Autodesk Fusion 360 part; units mm, degrees
(part 7 of 14)
  arc A1856 (48.735, 36.8717) -> (48.735, 37.1384) centre (48.735, 37.005) ccw
  line L3081 (47.395, 52.0775) -> (47.395, 54.3505)
  line L3082 (46.395, 46.3495) -> (46.395, 48.6225)
  line L3083 (46.895, 52.0775) -> (46.895, 54.3505)
  line L3084 (17.461, 23.167) -> (27.461, 23.167)
  line L3085 (27.461, 13.167) -> (17.461, 13.167)
  arc A1857 (52.735, 36.8717) -> (52.735, 37.1384) centre (52.735, 37.005) ccw
  line L3086 (17.461, 13.167) -> (17.461, 23.167)
  line L3087 (61.3283, 55.098) -> (60.4393, 55.098)
  arc A1858 (16.7662, 22.5764) -> (17.1475, 22.5764) centre (16.9568, 22.5764) ccw
  arc A1859 (17.1475, 22.5764) -> (16.7662, 22.5764) centre (16.9568, 22.5764) ccw
  line L3088 (27.461, 23.167) -> (27.461, 13.167)
  arc A1860 (50.735, 37.1384) -> (50.735, 36.8717) centre (50.735, 37.005) ccw
  line L3089 (46.395, 46.3495) -> (46.395, 48.6225)
  line L3090 (46.895, 46.3495) -> (46.895, 48.6225)
  line L3091 (47.395, 46.3495) -> (47.395, 48.6225)
  line L3092 (47.895, 46.3495) -> (47.895, 48.6225)
  arc A1861 (51.735, 36.8717) -> (51.735, 37.1384) centre (51.735, 37.005) ccw
  arc A1862 (49.735, 36.8717) -> (49.735, 37.1384) centre (49.735, 37.005) ccw
  arc A1863 (52.735, 36.8717) -> (52.735, 37.1384) centre (52.735, 37.005) ccw
  arc A1864 (50.735, 36.8717) -> (50.735, 37.1384) centre (50.735, 37.005) ccw
  arc A1865 (51.735, 37.1384) -> (51.735, 36.8717) centre (51.735, 37.005) ccw
  arc A1866 (48.735, 36.8717) -> (48.735, 37.1384) centre (48.735, 37.005) ccw
  arc A1867 (52.735, 36.8717) -> (52.735, 37.1384) centre (52.735, 37.005) ccw
  arc A1868 (50.735, 37.1384) -> (50.735, 36.8717) centre (50.735, 37.005) ccw
  arc A1869 (51.735, 36.8717) -> (51.735, 37.1384) centre (51.735, 37.005) ccw
  arc A1870 (51.735, 37.1384) -> (51.735, 36.8717) centre (51.735, 37.005) ccw
  arc A1871 (51.735, 37.1384) -> (51.735, 36.8717) centre (51.735, 37.005) ccw
  arc A1872 (50.735, 37.1384) -> (50.735, 36.8717) centre (50.735, 37.005) ccw
  arc A1873 (48.735, 37.1384) -> (48.735, 36.8717) centre (48.735, 37.005) ccw
  arc A1874 (52.735, 37.1384) -> (52.735, 36.8717) centre (52.735, 37.005) ccw
  line L3093 (47.395, 52.0775) -> (47.395, 54.3505)
  line L3094 (47.895, 52.0775) -> (47.895, 54.3505)
  line L3095 (46.895, 46.3495) -> (46.895, 48.6225)
  line L3096 (47.395, 46.3495) -> (47.395, 48.6225)
  arc A1875 (50.735, 36.8717) -> (50.735, 37.1384) centre (50.735, 37.005) ccw
  line L3097 (47.895, 46.3495) -> (47.895, 48.6225)
  arc A1876 (49.735, 37.1384) -> (49.735, 36.8717) centre (49.735, 37.005) ccw
  line L3098 (46.895, 52.0775) -> (46.895, 54.3505)
  line L3099 (46.895, 46.3495) -> (46.895, 48.6225)
  line L3100 (47.895, 52.0775) -> (47.895, 54.3505)
  arc A1877 (49.735, 36.8717) -> (49.735, 37.1384) centre (49.735, 37.005) ccw
  line L3101 (47.27, 11.525) -> (45.492, 11.525)
  line L3102 (9.7348, 30.754) -> (9.7348, 30.246)
  line L3103 (0.0248, 38.77) -> (0.0248, 25.27)
  line L3104 (9.4808, 30.5) -> (9.9888, 30.5)
  line L3105 (-5.0452, 28.845) -> (-3.9452, 27.745)
  line L3106 (51.715, 9.112) -> (51.715, 15.081)
  line L3107 (47.905, 15.081) -> (47.905, 9.112)
  line L3108 (47.27, 9.112) -> (47.27, 15.081)
  line L3109 (47.27, 14.065) -> (45.492, 14.065)
  line L3110 (9.4808, 30.5) -> (9.9888, 30.5)
  arc A1878 (9.7348, 30.7477) -> (9.7348, 30.2524) centre (9.7348, 30.5) ccw
  line L3111 (-5.2752, 25.77) -> (4.9948, 25.77)
  line L3112 (9.7348, 30.754) -> (9.7348, 30.246)
  arc A1879 (9.7348, 30.2524) -> (9.7348, 30.7477) centre (9.7348, 30.5) ccw
  line L3113 (50.445, 9.747) -> (50.445, 10.382)
  line L3114 (51.715, 15.081) -> (47.905, 15.081)
  line L3115 (54.128, 11.525) -> (52.35, 11.525)
  arc A1880 (9.7348, 30.2524) -> (9.7348, 30.7477) centre (9.7348, 30.5) ccw
  line L3116 (54.128, 11.525) -> (52.35, 11.525)
  line L3117 (54.128, 12.795) -> (52.35, 12.795)
  line L3118 (9.7348, 30.754) -> (9.7348, 30.246)
  line L3119 (52.35, 15.081) -> (52.35, 9.112)
  line L3120 (49.81, 9.112) -> (47.27, 9.112)
  line L3121 (47.27, 14.065) -> (45.492, 14.065)
  line L3122 (9.4808, 30.5) -> (9.9888, 30.5)
  line L3123 (47.27, 15.081) -> (52.35, 15.081)
  line L3124 (13.0848, 25.77) -> (13.0848, 37.77)
  line L3125 (9.7348, 30.754) -> (9.7348, 30.246)
  line L3126 (52.35, 9.112) -> (49.81, 9.112)
  line L3127 (47.905, 9.112) -> (51.715, 9.112)
  arc A1881 (9.7348, 30.7477) -> (9.7348, 30.2524) centre (9.7348, 30.5) ccw
  line L3128 (4.7648, 37.77) -> (-5.2752, 37.77)
  line L3129 (47.27, 11.525) -> (45.492, 11.525)
  arc A1882 (9.7348, 30.2524) -> (9.7348, 30.7477) centre (9.7348, 30.5) ccw
  arc A1883 (9.7348, 30.2524) -> (9.7348, 30.7477) centre (9.7348, 30.5) ccw
  line L3130 (54.128, 10.255) -> (52.35, 10.255)
  line L3131 (54.128, 11.525) -> (52.35, 11.525)
  line L3132 (54.128, 10.255) -> (52.35, 10.255)
  line L3133 (51.715, 9.747) -> (50.445, 9.747)
  line L3134 (54.128, 12.795) -> (52.35, 12.795)
  line L3135 (51.715, 9.112) -> (51.715, 15.081)
  line L3136 (50.445, 10.382) -> (51.715, 10.382)
  line L3137 (54.128, 14.065) -> (52.35, 14.065)
  line L3138 (54.128, 10.255) -> (52.35, 10.255)
  arc A1884 (9.7348, 30.7477) -> (9.7348, 30.2524) centre (9.7348, 30.5) ccw
  arc A1885 (53.747, 8.477) -> (52.985, 8.477) centre (53.366, 8.477) ccw
  line L3139 (54.128, 12.795) -> (52.35, 12.795)
  line L3140 (47.27, 11.525) -> (45.492, 11.525)
  arc A1886 (9.7348, 30.2524) -> (9.7348, 30.7477) centre (9.7348, 30.5) ccw
  arc A1887 (9.7348, 30.7477) -> (9.7348, 30.2524) centre (9.7348, 30.5) ccw
  line L3141 (-5.2752, 37.77) -> (-5.2752, 25.77)
  line L3142 (54.128, 14.065) -> (52.35, 14.065)
  line L3143 (-3.9452, 27.745) -> (-5.1452, 26.545)
  line L3144 (9.7348, 30.754) -> (9.7348, 30.246)
  arc A1888 (9.7348, 30.7477) -> (9.7348, 30.2524) centre (9.7348, 30.5) ccw
  line L3145 (47.27, 10.255) -> (45.492, 10.255)
  arc A1889 (9.7348, 30.2524) -> (9.7348, 30.7477) centre (9.7348, 30.5) ccw
  line L3146 (47.27, 14.065) -> (45.492, 14.065)
  line L3147 (9.4808, 30.5) -> (9.9888, 30.5)
  line L3148 (9.4808, 30.5) -> (9.9888, 30.5)
  arc A1890 (52.985, 8.477) -> (53.747, 8.477) centre (53.366, 8.477) ccw
  line L3149 (47.27, 12.795) -> (45.492, 12.795)
  line L3150 (54.128, 14.065) -> (52.35, 14.065)
  arc A1891 (9.7348, 30.7477) -> (9.7348, 30.2524) centre (9.7348, 30.5) ccw
  line L3151 (9.7348, 30.754) -> (9.7348, 30.246)
  arc A1892 (10.1158, 30.5) -> (9.3538, 30.5) centre (9.7348, 30.5) ccw
  arc A1893 (9.3538, 30.5) -> (10.1158, 30.5) centre (9.7348, 30.5) ccw
  arc A1894 (9.7348, 33.2476) -> (9.7348, 32.7523) centre (9.7348, 33) ccw
  line L3152 (9.4808, 33) -> (9.9888, 33)
  arc A1895 (9.7348, 33.2476) -> (9.7348, 32.7523) centre (9.7348, 33) ccw
  arc A1896 (9.7348, 30.7477) -> (9.7348, 30.2524) centre (9.7348, 30.5) ccw
  arc A1897 (9.7348, 30.7477) -> (9.7348, 30.2524) centre (9.7348, 30.5) ccw
  line L3153 (47.27, 12.795) -> (45.492, 12.795)
  arc A1898 (9.7348, 33.2476) -> (9.7348, 32.7523) centre (9.7348, 33) ccw
  line L3154 (47.27, 10.255) -> (45.492, 10.255)
  arc A1899 (9.7348, 32.7523) -> (9.7348, 33.2476) centre (9.7348, 33) ccw
  arc A1900 (9.7348, 30.2524) -> (9.7348, 30.7477) centre (9.7348, 30.5) ccw
  line L3155 (9.4808, 30.5) -> (9.9888, 30.5)
  arc A1901 (9.7348, 32.7523) -> (9.7348, 33.2476) centre (9.7348, 33) ccw
  line L3156 (9.4808, 33) -> (9.9888, 33)
  arc A1902 (9.7348, 32.7523) -> (9.7348, 33.2476) centre (9.7348, 33) ccw
  arc A1903 (9.7348, 32.7523) -> (9.7348, 33.2476) centre (9.7348, 33) ccw
  line L3157 (9.7348, 33.254) -> (9.7348, 32.746)
  line L3158 (9.7348, 30.754) -> (9.7348, 30.246)
  line L3159 (9.4808, 33) -> (9.9888, 33)
  line L3160 (47.27, 12.795) -> (45.492, 12.795)
  line L3161 (9.7348, 30.754) -> (9.7348, 30.246)
  line L3162 (4.7648, 25.77) -> (13.0848, 25.77)
  arc A1904 (9.7348, 33.2476) -> (9.7348, 32.7523) centre (9.7348, 33) ccw
  line L3163 (9.7348, 33.254) -> (9.7348, 32.746)
  arc A1905 (9.7348, 30.7477) -> (9.7348, 30.2524) centre (9.7348, 30.5) ccw
  line L3164 (9.7348, 33.254) -> (9.7348, 32.746)
  arc A1906 (9.7348, 30.2524) -> (9.7348, 30.7477) centre (9.7348, 30.5) ccw
  arc A1907 (9.7348, 30.2524) -> (9.7348, 30.7477) centre (9.7348, 30.5) ccw
  arc A1908 (10.1158, 30.5) -> (9.3538, 30.5) centre (9.7348, 30.5) ccw
  arc A1909 (9.7348, 33.2476) -> (9.7348, 32.7523) centre (9.7348, 33) ccw
  line L3165 (9.4808, 30.5) -> (9.9888, 30.5)
  line L3166 (9.4808, 33) -> (9.9888, 33)
  arc A1910 (9.7348, 33.2476) -> (9.7348, 32.7523) centre (9.7348, 33) ccw
  arc A1911 (9.7348, 33.2476) -> (9.7348, 32.7523) centre (9.7348, 33) ccw
  line L3167 (9.4808, 33) -> (9.9888, 33)
  arc A1912 (9.3538, 30.5) -> (10.1158, 30.5) centre (9.7348, 30.5) ccw
  line L3168 (9.4808, 30.5) -> (9.9888, 30.5)
  line L3169 (9.7348, 33.254) -> (9.7348, 32.746)
  arc A1913 (9.7348, 33.2476) -> (9.7348, 32.7523) centre (9.7348, 33) ccw
  arc A1914 (9.7348, 30.7477) -> (9.7348, 30.2524) centre (9.7348, 30.5) ccw
  line L3170 (9.7348, 30.754) -> (9.7348, 30.246)
  line L3171 (13.0848, 37.77) -> (4.7648, 37.77)
  line L3172 (9.7348, 33.254) -> (9.7348, 32.746)
  line L3173 (9.7348, 33.254) -> (9.7348, 32.746)
  arc A1915 (9.7348, 32.7523) -> (9.7348, 33.2476) centre (9.7348, 33) ccw
  line L3174 (9.4808, 30.5) -> (9.9888, 30.5)
  arc A1916 (10.1158, 30.5) -> (9.3538, 30.5) centre (9.7348, 30.5) ccw
  arc A1917 (9.7348, 32.7523) -> (9.7348, 33.2476) centre (9.7348, 33) ccw
  arc A1918 (9.3538, 30.5) -> (10.1158, 30.5) centre (9.7348, 30.5) ccw
  line L3175 (9.7348, 33.254) -> (9.7348, 32.746)
  line L3176 (9.4808, 33) -> (9.9888, 33)
  line L3177 (9.4808, 30.5) -> (9.9888, 30.5)
  arc A1919 (9.7348, 32.7523) -> (9.7348, 33.2476) centre (9.7348, 33) ccw
  arc A1920 (9.3538, 30.5) -> (10.1158, 30.5) centre (9.7348, 30.5) ccw
  arc A1921 (9.7348, 33.2476) -> (9.7348, 32.7523) centre (9.7348, 33) ccw
  line L3178 (47.27, 10.255) -> (45.492, 10.255)
  arc A1922 (10.1158, 30.5) -> (9.3538, 30.5) centre (9.7348, 30.5) ccw
  arc A1923 (9.7348, 30.2524) -> (9.7348, 30.7477) centre (9.7348, 30.5) ccw
  line L3179 (9.4808, 33) -> (9.9888, 33)
  arc A1924 (10.1158, 30.5) -> (9.3538, 30.5) centre (9.7348, 30.5) ccw
  line L3180 (9.7348, 30.754) -> (9.7348, 30.246)
  arc A1925 (9.7348, 33.2476) -> (9.7348, 32.7523) centre (9.7348, 33) ccw
  line L3181 (9.7348, 33.254) -> (9.7348, 32.746)
  line L3182 (7.4808, 33) -> (7.9888, 33)
  arc A1926 (7.7348, 32.7523) -> (7.7348, 33.2476) centre (7.7348, 33) ccw
  line L3183 (7.7348, 33.254) -> (7.7348, 32.746)
  line L3184 (7.7348, 33.254) -> (7.7348, 32.746)
  arc A1927 (10.1158, 33) -> (9.3538, 33) centre (9.7348, 33) ccw
  arc A1928 (7.7348, 33.2476) -> (7.7348, 32.7523) centre (7.7348, 33) ccw
  arc A1929 (7.7348, 33.2476) -> (7.7348, 32.7523) centre (7.7348, 33) ccw
  line L3185 (7.4808, 33) -> (7.9888, 33)
  arc A1930 (9.3538, 33) -> (10.1158, 33) centre (9.7348, 33) ccw
  arc A1931 (10.1158, 33) -> (9.3538, 33) centre (9.7348, 33) ccw
  arc A1932 (7.7348, 33.2476) -> (7.7348, 32.7523) centre (7.7348, 33) ccw
  arc A1933 (10.1158, 33) -> (9.3538, 33) centre (9.7348, 33) ccw
  line L3186 (7.7348, 33.254) -> (7.7348, 32.746)
  line L3187 (7.4808, 33) -> (7.9888, 33)
  line L3188 (9.4808, 33) -> (9.9888, 33)
  arc A1934 (9.3538, 33) -> (10.1158, 33) centre (9.7348, 33) ccw
  line L3189 (7.7348, 33.254) -> (7.7348, 32.746)
  arc A1935 (7.7348, 32.7523) -> (7.7348, 33.2476) centre (7.7348, 33) ccw
  arc A1936 (7.7348, 32.7523) -> (7.7348, 33.2476) centre (7.7348, 33) ccw
  line L3190 (7.7348, 33.254) -> (7.7348, 32.746)
  line L3191 (9.4808, 33) -> (9.9888, 33)
  line L3192 (7.7348, 33.254) -> (7.7348, 32.746)
  line L3193 (7.4808, 33) -> (7.9888, 33)
  arc A1937 (8.1158, 33) -> (7.3538, 33) centre (7.7348, 33) ccw
  arc A1938 (7.7348, 33.2476) -> (7.7348, 32.7523) centre (7.7348, 33) ccw
  arc A1939 (7.7348, 33.2476) -> (7.7348, 32.7523) centre (7.7348, 33) ccw
  arc A1940 (7.3538, 33) -> (8.1158, 33) centre (7.7348, 33) ccw
  arc A1941 (10.1158, 33) -> (9.3538, 33) centre (9.7348, 33) ccw
  arc A1942 (7.7348, 32.7523) -> (7.7348, 33.2476) centre (7.7348, 33) ccw
  arc A1943 (7.7348, 32.7523) -> (7.7348, 33.2476) centre (7.7348, 33) ccw
  line L3194 (7.4808, 33) -> (7.9888, 33)
  line L3195 (7.7348, 33.254) -> (7.7348, 32.746)
  arc A1944 (9.3538, 33) -> (10.1158, 33) centre (9.7348, 33) ccw
  arc A1945 (7.7348, 32.7523) -> (7.7348, 33.2476) centre (7.7348, 33) ccw
  line L3196 (7.7348, 33.254) -> (7.7348, 32.746)
  arc A1946 (7.3538, 33) -> (8.1158, 33) centre (7.7348, 33) ccw
  line L3197 (7.4808, 33) -> (7.9888, 33)
  line L3198 (7.7348, 33.254) -> (7.7348, 32.746)
  line L3199 (7.4808, 33) -> (7.9888, 33)
  arc A1947 (7.7348, 32.7523) -> (7.7348, 33.2476) centre (7.7348, 33) ccw
  arc A1948 (9.3538, 33) -> (10.1158, 33) centre (9.7348, 33) ccw
  line L3200 (7.4808, 33) -> (7.9888, 33)
  line L3201 (9.7348, 33.254) -> (9.7348, 32.746)
  line L3202 (9.7348, 33.254) -> (9.7348, 32.746)
  arc A1949 (9.7348, 32.7523) -> (9.7348, 33.2476) centre (9.7348, 33) ccw
  line L3203 (9.4808, 33) -> (9.9888, 33)
  arc A1950 (9.3538, 30.5) -> (10.1158, 30.5) centre (9.7348, 30.5) ccw
  arc A1951 (7.7348, 33.2476) -> (7.7348, 32.7523) centre (7.7348, 33) ccw
  arc A1952 (7.7348, 32.7523) -> (7.7348, 33.2476) centre (7.7348, 33) ccw
  arc A1953 (9.3538, 33) -> (10.1158, 33) centre (9.7348, 33) ccw
  line L3204 (7.7348, 33.254) -> (7.7348, 32.746)
  arc A1954 (9.7348, 32.7523) -> (9.7348, 33.2476) centre (9.7348, 33) ccw
  arc A1955 (9.7348, 32.7523) -> (9.7348, 33.2476) centre (9.7348, 33) ccw
  arc A1956 (7.7348, 32.7523) -> (7.7348, 33.2476) centre (7.7348, 33) ccw
  arc A1957 (7.7348, 33.2476) -> (7.7348, 32.7523) centre (7.7348, 33) ccw
  arc A1958 (10.1158, 33) -> (9.3538, 33) centre (9.7348, 33) ccw
  arc A1959 (7.3538, 33) -> (8.1158, 33) centre (7.7348, 33) ccw
  line L3205 (7.4808, 33) -> (7.9888, 33)
  arc A1960 (7.7348, 33.2476) -> (7.7348, 32.7523) centre (7.7348, 33) ccw
  arc A1961 (7.7348, 32.7523) -> (7.7348, 33.2476) centre (7.7348, 33) ccw
  arc A1962 (7.7348, 33.2476) -> (7.7348, 32.7523) centre (7.7348, 33) ccw
  line L3206 (7.4808, 33) -> (7.9888, 33)
  arc A1963 (7.7348, 33.2476) -> (7.7348, 32.7523) centre (7.7348, 33) ccw
  arc A1964 (11.7348, 35.7968) -> (11.7348, 36.2032) centre (11.7348, 36) ccw
  arc A1965 (11.7348, 35.7968) -> (11.7348, 36.2032) centre (11.7348, 36) ccw
  line L3207 (11.7348, 36.254) -> (11.7348, 35.746)
  line L3208 (7.4808, 30.5) -> (7.9888, 30.5)
  arc A1966 (11.7348, 34.0468) -> (11.7348, 34.4532) centre (11.7348, 34.25) ccw
  line L3209 (7.7348, 30.754) -> (7.7348, 30.246)
  arc A1967 (7.3538, 30.5) -> (8.1158, 30.5) centre (7.7348, 30.5) ccw
  arc A1968 (8.1158, 33) -> (7.3538, 33) centre (7.7348, 33) ccw
  line L3210 (7.4808, 30.5) -> (7.9888, 30.5)
  line L3211 (7.4808, 30.5) -> (7.9888, 30.5)
  arc A1969 (7.7348, 30.7477) -> (7.7348, 30.2524) centre (7.7348, 30.5) ccw
  arc A1970 (11.7348, 36.2032) -> (11.7348, 35.7968) centre (11.7348, 36) ccw
  line L3212 (11.4808, 36) -> (11.9888, 36)
  line L3213 (11.7348, 36.254) -> (11.7348, 35.746)
  arc A1971 (7.7348, 30.2524) -> (7.7348, 30.7477) centre (7.7348, 30.5) ccw
  arc A1972 (7.7348, 30.2524) -> (7.7348, 30.7477) centre (7.7348, 30.5) ccw
  arc A1973 (7.7348, 30.2524) -> (7.7348, 30.7477) centre (7.7348, 30.5) ccw
  arc A1974 (7.3538, 33) -> (8.1158, 33) centre (7.7348, 33) ccw
  arc A1975 (7.7348, 30.2524) -> (7.7348, 30.7477) centre (7.7348, 30.5) ccw
  line L3214 (7.4808, 30.5) -> (7.9888, 30.5)
  arc A1976 (7.7348, 30.7477) -> (7.7348, 30.2524) centre (7.7348, 30.5) ccw
  line L3215 (7.7348, 30.754) -> (7.7348, 30.246)
  line L3216 (7.7348, 30.754) -> (7.7348, 30.246)
  arc A1977 (7.7348, 30.7477) -> (7.7348, 30.2524) centre (7.7348, 30.5) ccw
  arc A1978 (7.7348, 30.2524) -> (7.7348, 30.7477) centre (7.7348, 30.5) ccw
  arc A1979 (8.1158, 33) -> (7.3538, 33) centre (7.7348, 33) ccw
  line L3217 (7.4808, 30.5) -> (7.9888, 30.5)
  arc A1980 (7.3538, 30.5) -> (8.1158, 30.5) centre (7.7348, 30.5) ccw
  arc A1981 (7.3538, 33) -> (8.1158, 33) centre (7.7348, 33) ccw
  arc A1982 (7.7348, 30.2524) -> (7.7348, 30.7477) centre (7.7348, 30.5) ccw
  arc A1983 (8.1158, 30.5) -> (7.3538, 30.5) centre (7.7348, 30.5) ccw
  arc A1984 (8.1158, 30.5) -> (7.3538, 30.5) centre (7.7348, 30.5) ccw
  line L3218 (7.7348, 30.754) -> (7.7348, 30.246)
  line L3219 (7.4808, 30.5) -> (7.9888, 30.5)
  arc A1985 (7.7348, 30.7477) -> (7.7348, 30.2524) centre (7.7348, 30.5) ccw
  line L3220 (7.7348, 30.754) -> (7.7348, 30.246)
  arc A1986 (7.7348, 30.2524) -> (7.7348, 30.7477) centre (7.7348, 30.5) ccw
  line L3221 (7.7348, 30.754) -> (7.7348, 30.246)
  line L3222 (7.4808, 30.5) -> (7.9888, 30.5)
  arc A1987 (7.7348, 30.2524) -> (7.7348, 30.7477) centre (7.7348, 30.5) ccw
  arc A1988 (7.7348, 30.7477) -> (7.7348, 30.2524) centre (7.7348, 30.5) ccw
  arc A1989 (7.7348, 30.7477) -> (7.7348, 30.2524) centre (7.7348, 30.5) ccw
  arc A1990 (7.7348, 30.7477) -> (7.7348, 30.2524) centre (7.7348, 30.5) ccw
  arc A1991 (7.3538, 30.5) -> (8.1158, 30.5) centre (7.7348, 30.5) ccw
  line L3223 (7.7348, 30.754) -> (7.7348, 30.246)
  arc A1992 (7.7348, 30.2524) -> (7.7348, 30.7477) centre (7.7348, 30.5) ccw
  arc A1993 (8.1158, 30.5) -> (7.3538, 30.5) centre (7.7348, 30.5) ccw
  line L3224 (7.4808, 30.5) -> (7.9888, 30.5)
  arc A1994 (7.7348, 30.7477) -> (7.7348, 30.2524) centre (7.7348, 30.5) ccw
  line L3225 (7.7348, 30.754) -> (7.7348, 30.246)
  arc A1995 (8.1158, 33) -> (7.3538, 33) centre (7.7348, 33) ccw
  arc A1996 (7.3538, 30.5) -> (8.1158, 30.5) centre (7.7348, 30.5) ccw
  arc A1997 (7.7348, 30.7477) -> (7.7348, 30.2524) centre (7.7348, 30.5) ccw
  arc A1998 (7.7348, 30.2524) -> (7.7348, 30.7477) centre (7.7348, 30.5) ccw
  arc A1999 (8.1158, 30.5) -> (7.3538, 30.5) centre (7.7348, 30.5) ccw
  arc A2000 (7.7348, 30.7477) -> (7.7348, 30.2524) centre (7.7348, 30.5) ccw
  line L3226 (7.4808, 30.5) -> (7.9888, 30.5)
  line L3227 (7.4808, 30.5) -> (7.9888, 30.5)
  line L3228 (7.7348, 30.754) -> (7.7348, 30.246)
  arc A2001 (11.7348, 35.7968) -> (11.7348, 36.2032) centre (11.7348, 36) ccw
  line L3229 (7.7348, 30.754) -> (7.7348, 30.246)
  line L3230 (11.4808, 36) -> (11.9888, 36)
  arc A2002 (8.1158, 33) -> (7.3538, 33) centre (7.7348, 33) ccw
  arc A2003 (12.0523, 36) -> (11.4173, 36) centre (11.7348, 36) ccw
  arc A2004 (7.3538, 30.5) -> (8.1158, 30.5) centre (7.7348, 30.5) ccw
  line L3231 (11.7348, 36.254) -> (11.7348, 35.746)
  line L3232 (11.7348, 36.254) -> (11.7348, 35.746)
  line L3233 (11.4808, 36) -> (11.9888, 36)
  line L3234 (11.4808, 34.25) -> (11.9888, 34.25)
  arc A2005 (11.4173, 34.25) -> (12.0523, 34.25) centre (11.7348, 34.25) ccw
  line L3235 (11.7348, 34.504) -> (11.7348, 33.996)
  arc A2006 (11.7348, 36.2032) -> (11.7348, 35.7968) centre (11.7348, 36) ccw
  line L3236 (11.7348, 34.504) -> (11.7348, 33.996)
  arc A2007 (11.4173, 36) -> (12.0523, 36) centre (11.7348, 36) ccw
  arc A2008 (11.7348, 34.4532) -> (11.7348, 34.0468) centre (11.7348, 34.25) ccw
  arc A2009 (11.7348, 35.7968) -> (11.7348, 36.2032) centre (11.7348, 36) ccw
  line L3237 (11.4808, 36) -> (11.9888, 36)
  arc A2010 (11.4173, 36) -> (12.0523, 36) centre (11.7348, 36) ccw
  arc A2011 (11.7348, 36.2032) -> (11.7348, 35.7968) centre (11.7348, 36) ccw
  arc A2012 (11.7348, 34.0468) -> (11.7348, 34.4532) centre (11.7348, 34.25) ccw
  arc A2013 (12.0523, 36) -> (11.4173, 36) centre (11.7348, 36) ccw
  arc A2014 (11.7348, 35.7968) -> (11.7348, 36.2032) centre (11.7348, 36) ccw
  line L3238 (11.7348, 34.504) -> (11.7348, 33.996)
  line L3239 (11.4808, 36) -> (11.9888, 36)
  arc A2015 (11.7348, 34.0468) -> (11.7348, 34.4532) centre (11.7348, 34.25) ccw
  arc A2016 (11.7348, 34.0468) -> (11.7348, 34.4532) centre (11.7348, 34.25) ccw
  line L3240 (11.4808, 34.25) -> (11.9888, 34.25)
  arc A2017 (11.7348, 36.2032) -> (11.7348, 35.7968) centre (11.7348, 36) ccw
  line L3241 (11.7348, 34.504) -> (11.7348, 33.996)
  arc A2018 (11.7348, 34.4532) -> (11.7348, 34.0468) centre (11.7348, 34.25) ccw
  line L3242 (11.7348, 34.504) -> (11.7348, 33.996)
  arc A2019 (11.7348, 31.9532) -> (11.7348, 31.5468) centre (11.7348, 31.75) ccw
  arc A2020 (11.7348, 34.0468) -> (11.7348, 34.4532) centre (11.7348, 34.25) ccw
  line L3243 (11.4808, 34.25) -> (11.9888, 34.25)
  arc A2021 (11.7348, 34.0468) -> (11.7348, 34.4532) centre (11.7348, 34.25) ccw
  arc A2022 (11.7348, 35.7968) -> (11.7348, 36.2032) centre (11.7348, 36) ccw
  line L3244 (11.7348, 36.254) -> (11.7348, 35.746)
  arc A2023 (11.7348, 34.4532) -> (11.7348, 34.0468) centre (11.7348, 34.25) ccw
  arc A2024 (11.7348, 34.0468) -> (11.7348, 34.4532) centre (11.7348, 34.25) ccw
  arc A2025 (11.7348, 36.2032) -> (11.7348, 35.7968) centre (11.7348, 36) ccw
  arc A2026 (11.7348, 36.2032) -> (11.7348, 35.7968) centre (11.7348, 36) ccw
  line L3245 (11.4808, 36) -> (11.9888, 36)
  arc A2027 (8.1158, 30.5) -> (7.3538, 30.5) centre (7.7348, 30.5) ccw
  arc A2028 (11.7348, 36.2032) -> (11.7348, 35.7968) centre (11.7348, 36) ccw
  line L3246 (11.4808, 36) -> (11.9888, 36)
  arc A2029 (11.4173, 36) -> (12.0523, 36) centre (11.7348, 36) ccw
  line L3247 (11.7348, 36.254) -> (11.7348, 35.746)
  arc A2030 (11.7348, 34.4532) -> (11.7348, 34.0468) centre (11.7348, 34.25) ccw
  arc A2031 (11.7348, 35.7968) -> (11.7348, 36.2032) centre (11.7348, 36) ccw
  line L3248 (11.7348, 36.254) -> (11.7348, 35.746)
  arc A2032 (11.7348, 35.7968) -> (11.7348, 36.2032) centre (11.7348, 36) ccw
  arc A2033 (11.7348, 36.2032) -> (11.7348, 35.7968) centre (11.7348, 36) ccw
  arc A2034 (12.0523, 36) -> (11.4173, 36) centre (11.7348, 36) ccw
  line L3249 (11.7348, 36.254) -> (11.7348, 35.746)
  arc A2035 (12.0523, 36) -> (11.4173, 36) centre (11.7348, 36) ccw
  line L3250 (11.7348, 34.504) -> (11.7348, 33.996)
  line L3251 (11.4808, 36) -> (11.9888, 36)
  line L3252 (11.7348, 36.254) -> (11.7348, 35.746)
  line L3253 (11.7348, 36.254) -> (11.7348, 35.746)
  arc A2036 (11.7348, 36.2032) -> (11.7348, 35.7968) centre (11.7348, 36) ccw
  arc A2037 (11.4173, 36) -> (12.0523, 36) centre (11.7348, 36) ccw
  arc A2038 (11.7348, 36.2032) -> (11.7348, 35.7968) centre (11.7348, 36) ccw
  arc A2039 (11.4173, 36) -> (12.0523, 36) centre (11.7348, 36) ccw
  line L3254 (11.4808, 36) -> (11.9888, 36)
  arc A2040 (11.7348, 35.7968) -> (11.7348, 36.2032) centre (11.7348, 36) ccw
  arc A2041 (11.7348, 35.7968) -> (11.7348, 36.2032) centre (11.7348, 36) ccw
  line L3255 (11.4808, 36) -> (11.9888, 36)
  arc A2042 (12.0523, 36) -> (11.4173, 36) centre (11.7348, 36) ccw
  arc A2043 (12.0523, 31.75) -> (11.4173, 31.75) centre (11.7348, 31.75) ccw
  arc A2044 (11.7348, 34.0468) -> (11.7348, 34.4532) centre (11.7348, 34.25) ccw
  arc A2045 (12.0523, 31.75) -> (11.4173, 31.75) centre (11.7348, 31.75) ccw
  line L3256 (11.7348, 32.004) -> (11.7348, 31.496)
  line L3257 (11.7348, 32.004) -> (11.7348, 31.496)
  line L3258 (11.7348, 34.504) -> (11.7348, 33.996)
  line L3259 (11.7348, 32.004) -> (11.7348, 31.496)
  arc A2046 (11.7348, 31.9532) -> (11.7348, 31.5468) centre (11.7348, 31.75) ccw
  line L3260 (11.7348, 32.004) -> (11.7348, 31.496)
  arc A2047 (11.7348, 31.9532) -> (11.7348, 31.5468) centre (11.7348, 31.75) ccw
  arc A2048 (11.7348, 34.4532) -> (11.7348, 34.0468) centre (11.7348, 34.25) ccw
  line L3261 (11.4808, 34.25) -> (11.9888, 34.25)
  line L3262 (11.4808, 34.25) -> (11.9888, 34.25)
  line L3263 (11.7348, 32.004) -> (11.7348, 31.496)
  line L3264 (11.4808, 31.75) -> (11.9888, 31.75)
  arc A2049 (11.7348, 31.9532) -> (11.7348, 31.5468) centre (11.7348, 31.75) ccw
  arc A2050 (11.7348, 31.9532) -> (11.7348, 31.5468) centre (11.7348, 31.75) ccw
  arc A2051 (12.0523, 31.75) -> (11.4173, 31.75) centre (11.7348, 31.75) ccw
  arc A2052 (11.4173, 31.75) -> (12.0523, 31.75) centre (11.7348, 31.75) ccw
  arc A2053 (11.7348, 31.5468) -> (11.7348, 31.9532) centre (11.7348, 31.75) ccw
  arc A2054 (12.0523, 31.75) -> (11.4173, 31.75) centre (11.7348, 31.75) ccw
  line L3265 (11.4808, 31.75) -> (11.9888, 31.75)
  line L3266 (11.4808, 31.75) -> (11.9888, 31.75)
  line L3267 (11.4808, 34.25) -> (11.9888, 34.25)
  arc A2055 (11.7348, 29.4532) -> (11.7348, 29.0468) centre (11.7348, 29.25) ccw
  arc A2056 (11.7348, 29.4532) -> (11.7348, 29.0468) centre (11.7348, 29.25) ccw
  arc A2057 (11.7348, 29.0468) -> (11.7348, 29.4532) centre (11.7348, 29.25) ccw
  line L3268 (11.4808, 29.25) -> (11.9888, 29.25)
  arc A2058 (11.4173, 31.75) -> (12.0523, 31.75) centre (11.7348, 31.75) ccw
  arc A2059 (11.7348, 29.0468) -> (11.7348, 29.4532) centre (11.7348, 29.25) ccw
  arc A2060 (11.7348, 29.4532) -> (11.7348, 29.0468) centre (11.7348, 29.25) ccw
  arc A2061 (11.7348, 29.0468) -> (11.7348, 29.4532) centre (11.7348, 29.25) ccw
  line L3269 (11.7348, 29.504) -> (11.7348, 28.996)
  arc A2062 (11.7348, 31.5468) -> (11.7348, 31.9532) centre (11.7348, 31.75) ccw
  line L3270 (11.4808, 29.25) -> (11.9888, 29.25)
  arc A2063 (11.7348, 34.0468) -> (11.7348, 34.4532) centre (11.7348, 34.25) ccw
  arc A2064 (11.4173, 34.25) -> (12.0523, 34.25) centre (11.7348, 34.25) ccw
  line L3271 (11.4808, 31.75) -> (11.9888, 31.75)
  arc A2065 (11.4173, 34.25) -> (12.0523, 34.25) centre (11.7348, 34.25) ccw
  arc A2066 (12.0523, 34.25) -> (11.4173, 34.25) centre (11.7348, 34.25) ccw
  arc A2067 (11.7348, 34.4532) -> (11.7348, 34.0468) centre (11.7348, 34.25) ccw
  line L3272 (11.7348, 34.504) -> (11.7348, 33.996)
  line L3273 (11.7348, 34.504) -> (11.7348, 33.996)
  arc A2068 (11.7348, 34.0468) -> (11.7348, 34.4532) centre (11.7348, 34.25) ccw
  arc A2069 (12.0523, 34.25) -> (11.4173, 34.25) centre (11.7348, 34.25) ccw
  arc A2070 (11.7348, 34.4532) -> (11.7348, 34.0468) centre (11.7348, 34.25) ccw
  line L3274 (11.4808, 34.25) -> (11.9888, 34.25)
  arc A2071 (11.7348, 34.4532) -> (11.7348, 34.0468) centre (11.7348, 34.25) ccw
  arc A2072 (12.0523, 34.25) -> (11.4173, 34.25) centre (11.7348, 34.25) ccw
  arc A2073 (11.7348, 31.5468) -> (11.7348, 31.9532) centre (11.7348, 31.75) ccw
  arc A2074 (11.7348, 31.5468) -> (11.7348, 31.9532) centre (11.7348, 31.75) ccw
  line L3275 (11.7348, 34.504) -> (11.7348, 33.996)
  arc A2075 (11.7348, 34.4532) -> (11.7348, 34.0468) centre (11.7348, 34.25) ccw
  arc A2076 (12.0523, 34.25) -> (11.4173, 34.25) centre (11.7348, 34.25) ccw
  arc A2077 (11.4173, 34.25) -> (12.0523, 34.25) centre (11.7348, 34.25) ccw
  line L3276 (11.4808, 34.25) -> (11.9888, 34.25)
  line L3277 (11.7348, 32.004) -> (11.7348, 31.496)
  line L3278 (11.4808, 34.25) -> (11.9888, 34.25)
  arc A2078 (11.7348, 31.5468) -> (11.7348, 31.9532) centre (11.7348, 31.75) ccw
  line L3279 (11.4808, 31.75) -> (11.9888, 31.75)
  arc A2079 (12.0523, 34.25) -> (11.4173, 34.25) centre (11.7348, 34.25) ccw
  line L3280 (11.4808, 34.25) -> (11.9888, 34.25)
  arc A2080 (11.4173, 34.25) -> (12.0523, 34.25) centre (11.7348, 34.25) ccw
  arc A2081 (11.7348, 34.4532) -> (11.7348, 34.0468) centre (11.7348, 34.25) ccw
  arc A2082 (11.7348, 31.9532) -> (11.7348, 31.5468) centre (11.7348, 31.75) ccw
  arc A2083 (11.7348, 27.2768) -> (11.7348, 27.6832) centre (11.7348, 27.48) ccw
  arc A2084 (11.7348, 29.4532) -> (11.7348, 29.0468) centre (11.7348, 29.25) ccw
  line L3281 (11.7348, 27.734) -> (11.7348, 27.226)
  line L3282 (11.7348, 32.004) -> (11.7348, 31.496)
  arc A2085 (12.0523, 29.25) -> (11.4173, 29.25) centre (11.7348, 29.25) ccw
  arc A2086 (11.7348, 27.6832) -> (11.7348, 27.2768) centre (11.7348, 27.48) ccw
  arc A2087 (11.7348, 31.5468) -> (11.7348, 31.9532) centre (11.7348, 31.75) ccw
  arc A2088 (11.7348, 27.2768) -> (11.7348, 27.6832) centre (11.7348, 27.48) ccw
  arc A2089 (11.4173, 29.25) -> (12.0523, 29.25) centre (11.7348, 29.25) ccw
  line L3283 (11.4808, 27.48) -> (11.9888, 27.48)
  line L3284 (11.4808, 31.75) -> (11.9888, 31.75)
  arc A2090 (11.7348, 31.5468) -> (11.7348, 31.9532) centre (11.7348, 31.75) ccw
  arc A2091 (11.7348, 31.9532) -> (11.7348, 31.5468) centre (11.7348, 31.75) ccw
  line L3285 (11.7348, 29.504) -> (11.7348, 28.996)
  arc A2092 (11.7348, 31.9532) -> (11.7348, 31.5468) centre (11.7348, 31.75) ccw
  line L3286 (11.4808, 31.75) -> (11.9888, 31.75)
  arc A2093 (11.7348, 29.0468) -> (11.7348, 29.4532) centre (11.7348, 29.25) ccw
  line L3287 (11.4808, 29.25) -> (11.9888, 29.25)
  line L3288 (11.7348, 27.734) -> (11.7348, 27.226)
  line L3289 (11.7348, 32.004) -> (11.7348, 31.496)
  arc A2094 (11.7348, 29.0468) -> (11.7348, 29.4532) centre (11.7348, 29.25) ccw
  line L3290 (11.4808, 27.48) -> (11.9888, 27.48)
  arc A2095 (12.0523, 29.25) -> (11.4173, 29.25) centre (11.7348, 29.25) ccw
  arc A2096 (11.7348, 27.6832) -> (11.7348, 27.2768) centre (11.7348, 27.48) ccw
  line L3291 (11.7348, 29.504) -> (11.7348, 28.996)
  line L3292 (11.4808, 31.75) -> (11.9888, 31.75)
  arc A2097 (11.7348, 27.6832) -> (11.7348, 27.2768) centre (11.7348, 27.48) ccw
  arc A2098 (11.7348, 27.2768) -> (11.7348, 27.6832) centre (11.7348, 27.48) ccw
  line L3293 (11.4808, 29.25) -> (11.9888, 29.25)
  arc A2099 (11.7348, 31.5468) -> (11.7348, 31.9532) centre (11.7348, 31.75) ccw
  arc A2100 (11.4173, 31.75) -> (12.0523, 31.75) centre (11.7348, 31.75) ccw
  arc A2101 (11.7348, 31.5468) -> (11.7348, 31.9532) centre (11.7348, 31.75) ccw
  arc A2102 (11.7348, 29.4532) -> (11.7348, 29.0468) centre (11.7348, 29.25) ccw
  line L3294 (11.7348, 32.004) -> (11.7348, 31.496)
  line L3295 (11.4808, 31.75) -> (11.9888, 31.75)
  line L3296 (11.7348, 32.004) -> (11.7348, 31.496)
  line L3297 (11.7348, 29.504) -> (11.7348, 28.996)
  arc A2103 (11.7348, 31.9532) -> (11.7348, 31.5468) centre (11.7348, 31.75) ccw
  arc A2104 (11.7348, 27.2768) -> (11.7348, 27.6832) centre (11.7348, 27.48) ccw
  line L3298 (11.4808, 29.25) -> (11.9888, 29.25)
  arc A2105 (11.7348, 27.6832) -> (11.7348, 27.2768) centre (11.7348, 27.48) ccw
  arc A2106 (11.4173, 31.75) -> (12.0523, 31.75) centre (11.7348, 31.75) ccw
  arc A2107 (11.7348, 31.9532) -> (11.7348, 31.5468) centre (11.7348, 31.75) ccw
  line L3299 (11.4808, 29.25) -> (11.9888, 29.25)
  arc A2108 (11.7348, 27.2768) -> (11.7348, 27.6832) centre (11.7348, 27.48) ccw
  arc A2109 (11.7348, 27.6832) -> (11.7348, 27.2768) centre (11.7348, 27.48) ccw
  arc A2110 (11.7348, 29.4532) -> (11.7348, 29.0468) centre (11.7348, 29.25) ccw
  arc A2111 (12.0523, 29.25) -> (11.4173, 29.25) centre (11.7348, 29.25) ccw
  line L3300 (11.7348, 29.504) -> (11.7348, 28.996)
  arc A2112 (11.7348, 29.0468) -> (11.7348, 29.4532) centre (11.7348, 29.25) ccw
  line L3301 (11.4808, 31.75) -> (11.9888, 31.75)
  line L3302 (11.7348, 29.504) -> (11.7348, 28.996)
  arc A2113 (11.7348, 29.4532) -> (11.7348, 29.0468) centre (11.7348, 29.25) ccw
  arc A2114 (11.4173, 31.75) -> (12.0523, 31.75) centre (11.7348, 31.75) ccw
  line L3303 (11.7348, 29.504) -> (11.7348, 28.996)
  line L3304 (11.4808, 29.25) -> (11.9888, 29.25)
  arc A2115 (12.0523, 31.75) -> (11.4173, 31.75) centre (11.7348, 31.75) ccw
  arc A2116 (11.7348, 29.4532) -> (11.7348, 29.0468) centre (11.7348, 29.25) ccw
  line L3305 (11.4808, 29.25) -> (11.9888, 29.25)
  arc A2117 (11.7348, 31.5468) -> (11.7348, 31.9532) centre (11.7348, 31.75) ccw
  arc A2118 (11.7348, 29.4532) -> (11.7348, 29.0468) centre (11.7348, 29.25) ccw
  line L3306 (11.4808, 29.25) -> (11.9888, 29.25)
  line L3307 (11.7348, 29.504) -> (11.7348, 28.996)
  line L3308 (5.0248, 25.984) -> (5.0248, 25.476)
  line L3309 (5.0248, 25.984) -> (5.0248, 25.476)
  line L3310 (4.7708, 25.73) -> (5.2788, 25.73)
  arc A2119 (5.0248, 25.1395) -> (5.0248, 26.3206) centre (5.0248, 25.73) ccw
  arc A2120 (5.0248, 26.3206) -> (5.0248, 25.1395) centre (5.0248, 25.73) ccw
  line L3311 (5.0248, 25.984) -> (5.0248, 25.476)
  line L3312 (4.7708, 25.73) -> (5.2788, 25.73)
  line L3313 (11.4808, 27.48) -> (11.9888, 27.48)
  arc A2121 (11.4173, 27.48) -> (12.0523, 27.48) centre (11.7348, 27.48) ccw
  arc A2122 (11.4173, 27.48) -> (12.0523, 27.48) centre (11.7348, 27.48) ccw
  arc A2123 (11.7348, 29.4532) -> (11.7348, 29.0468) centre (11.7348, 29.25) ccw
  arc A2124 (11.7348, 27.2768) -> (11.7348, 27.6832) centre (11.7348, 27.48) ccw
  arc A2125 (5.0248, 26.3206) -> (5.0248, 25.1395) centre (5.0248, 25.73) ccw
  arc A2126 (5.0248, 26.3206) -> (5.0248, 25.1395) centre (5.0248, 25.73) ccw
  arc A2127 (11.4173, 27.48) -> (12.0523, 27.48) centre (11.7348, 27.48) ccw
  arc A2128 (11.7348, 29.0468) -> (11.7348, 29.4532) centre (11.7348, 29.25) ccw
  line L3314 (11.4808, 27.48) -> (11.9888, 27.48)
  arc A2129 (11.7348, 27.2768) -> (11.7348, 27.6832) centre (11.7348, 27.48) ccw
  line L3315 (11.4808, 27.48) -> (11.9888, 27.48)
  arc A2130 (11.4173, 29.25) -> (12.0523, 29.25) centre (11.7348, 29.25) ccw
  arc A2131 (12.0523, 29.25) -> (11.4173, 29.25) centre (11.7348, 29.25) ccw
  line L3316 (11.7348, 29.504) -> (11.7348, 28.996)
  arc A2132 (11.7348, 27.6832) -> (11.7348, 27.2768) centre (11.7348, 27.48) ccw
  arc A2133 (11.4173, 29.25) -> (12.0523, 29.25) centre (11.7348, 29.25) ccw
  arc A2134 (5.0248, 26.3206) -> (5.0248, 25.1395) centre (5.0248, 25.73) ccw
  arc A2135 (5.0248, 26.3206) -> (5.0248, 25.1395) centre (5.0248, 25.73) ccw
  line L3317 (11.4808, 27.48) -> (11.9888, 27.48)
  arc A2136 (12.0523, 27.48) -> (11.4173, 27.48) centre (11.7348, 27.48) ccw
  line L3318 (11.7348, 27.734) -> (11.7348, 27.226)
  arc A2137 (5.0248, 25.1395) -> (5.0248, 26.3206) centre (5.0248, 25.73) ccw
  line L3319 (11.7348, 27.734) -> (11.7348, 27.226)
  line L3320 (11.7348, 27.734) -> (11.7348, 27.226)
  line L3321 (4.7708, 25.73) -> (5.2788, 25.73)
  line L3322 (11.7348, 27.734) -> (11.7348, 27.226)
  arc A2138 (5.0248, 25.1395) -> (5.0248, 26.3206) centre (5.0248, 25.73) ccw
  line L3323 (11.7348, 27.734) -> (11.7348, 27.226)
  line L3324 (4.7708, 25.73) -> (5.2788, 25.73)
  arc A2139 (12.0523, 27.48) -> (11.4173, 27.48) centre (11.7348, 27.48) ccw
  arc A2140 (11.7348, 27.6832) -> (11.7348, 27.2768) centre (11.7348, 27.48) ccw
  arc A2141 (11.7348, 29.0468) -> (11.7348, 29.4532) centre (11.7348, 29.25) ccw
  line L3325 (4.7708, 25.73) -> (5.2788, 25.73)
  arc A2142 (11.7348, 29.0468) -> (11.7348, 29.4532) centre (11.7348, 29.25) ccw
  line L3326 (5.0248, 25.984) -> (5.0248, 25.476)
  line L3327 (11.4808, 27.48) -> (11.9888, 27.48)
  line L3328 (11.7348, 27.734) -> (11.7348, 27.226)
  arc A2143 (12.0523, 29.25) -> (11.4173, 29.25) centre (11.7348, 29.25) ccw
  line L3329 (11.7348, 27.734) -> (11.7348, 27.226)
  arc A2144 (5.0248, 26.3206) -> (5.0248, 25.1395) centre (5.0248, 25.73) ccw
  line L3330 (5.0248, 25.984) -> (5.0248, 25.476)
  arc A2145 (5.0248, 25.1395) -> (5.0248, 26.3206) centre (5.0248, 25.73) ccw
  line L3331 (4.7708, 25.73) -> (5.2788, 25.73)
  arc A2146 (11.4173, 29.25) -> (12.0523, 29.25) centre (11.7348, 29.25) ccw
  arc A2147 (11.4173, 29.25) -> (12.0523, 29.25) centre (11.7348, 29.25) ccw
  line L3332 (11.4808, 27.48) -> (11.9888, 27.48)
  line L3333 (11.7348, 29.504) -> (11.7348, 28.996)
  line L3334 (11.4808, 29.25) -> (11.9888, 29.25)
  line L3335 (11.4808, 27.48) -> (11.9888, 27.48)
  arc A2148 (11.4173, 27.48) -> (12.0523, 27.48) centre (11.7348, 27.48) ccw
  arc A2149 (11.7348, 27.6832) -> (11.7348, 27.2768) centre (11.7348, 27.48) ccw
  arc A2150 (11.7348, 27.6832) -> (11.7348, 27.2768) centre (11.7348, 27.48) ccw
  line L3336 (5.0248, 25.984) -> (5.0248, 25.476)
  arc A2151 (11.7348, 29.0468) -> (11.7348, 29.4532) centre (11.7348, 29.25) ccw
  arc A2152 (11.7348, 27.2768) -> (11.7348, 27.6832) centre (11.7348, 27.48) ccw
  arc A2153 (11.7348, 27.2768) -> (11.7348, 27.6832) centre (11.7348, 27.48) ccw
  arc A2154 (5.0248, 38.3605) -> (5.0248, 37.1794) centre (5.0248, 37.77) ccw
  arc A2155 (5.9138, 25.73) -> (4.1358, 25.73) centre (5.0248, 25.73) ccw
  line L3337 (4.7708, 37.77) -> (5.2788, 37.77)
  arc A2156 (5.9138, 25.73) -> (4.1358, 25.73) centre (5.0248, 25.73) ccw
  arc A2157 (5.9138, 25.73) -> (4.1358, 25.73) centre (5.0248, 25.73) ccw
  line L3338 (4.7708, 25.73) -> (5.2788, 25.73)
  arc A2158 (12.0523, 27.48) -> (11.4173, 27.48) centre (11.7348, 27.48) ccw
  arc A2159 (5.0248, 37.1794) -> (5.0248, 38.3605) centre (5.0248, 37.77) ccw
  line L3339 (4.7708, 37.77) -> (5.2788, 37.77)
  line L3340 (4.7708, 25.73) -> (5.2788, 25.73)
  line L3341 (4.7708, 37.77) -> (5.2788, 37.77)
  arc A2160 (5.9138, 25.73) -> (4.1358, 25.73) centre (5.0248, 25.73) ccw
  line L3342 (5.0248, 25.984) -> (5.0248, 25.476)
  arc A2161 (5.0248, 38.3605) -> (5.0248, 37.1794) centre (5.0248, 37.77) ccw
  arc A2162 (5.0248, 37.1794) -> (5.0248, 38.3605) centre (5.0248, 37.77) ccw
  arc A2163 (5.0248, 38.3605) -> (5.0248, 37.1794) centre (5.0248, 37.77) ccw
  arc A2164 (5.0248, 26.3206) -> (5.0248, 25.1395) centre (5.0248, 25.73) ccw
  arc A2165 (5.0248, 26.3206) -> (5.0248, 25.1395) centre (5.0248, 25.73) ccw
  arc A2166 (5.0248, 37.1794) -> (5.0248, 38.3605) centre (5.0248, 37.77) ccw
  arc A2167 (5.0248, 25.1395) -> (5.0248, 26.3206) centre (5.0248, 25.73) ccw
  line L3343 (4.7708, 25.73) -> (5.2788, 25.73)
  arc A2168 (5.0248, 38.3605) -> (5.0248, 37.1794) centre (5.0248, 37.77) ccw
  arc A2169 (5.0248, 25.1395) -> (5.0248, 26.3206) centre (5.0248, 25.73) ccw
  line L3344 (5.0248, 38.024) -> (5.0248, 37.516)
  arc A2170 (5.0248, 38.3605) -> (5.0248, 37.1794) centre (5.0248, 37.77) ccw
  arc A2171 (4.1358, 25.73) -> (5.9138, 25.73) centre (5.0248, 25.73) ccw
  line L3345 (5.0248, 25.984) -> (5.0248, 25.476)
  line L3346 (5.0248, 38.024) -> (5.0248, 37.516)
  arc A2172 (5.0248, 26.3206) -> (5.0248, 25.1395) centre (5.0248, 25.73) ccw
  arc A2173 (5.0248, 37.1794) -> (5.0248, 38.3605) centre (5.0248, 37.77) ccw
  arc A2174 (5.0248, 38.3605) -> (5.0248, 37.1794) centre (5.0248, 37.77) ccw
  line L3347 (5.0248, 38.024) -> (5.0248, 37.516)
  arc A2175 (5.0248, 25.1395) -> (5.0248, 26.3206) centre (5.0248, 25.73) ccw
  arc A2176 (5.9138, 25.73) -> (4.1358, 25.73) centre (5.0248, 25.73) ccw
  line L3348 (5.0248, 25.984) -> (5.0248, 25.476)
  arc A2177 (5.0248, 38.3605) -> (5.0248, 37.1794) centre (5.0248, 37.77) ccw
  arc A2178 (5.0248, 38.3605) -> (5.0248, 37.1794) centre (5.0248, 37.77) ccw
  arc A2179 (5.0248, 38.3605) -> (5.0248, 37.1794) centre (5.0248, 37.77) ccw
  arc A2180 (4.1358, 25.73) -> (5.9138, 25.73) centre (5.0248, 25.73) ccw
  arc A2181 (5.0248, 25.1395) -> (5.0248, 26.3206) centre (5.0248, 25.73) ccw
  arc A2182 (5.0248, 25.1395) -> (5.0248, 26.3206) centre (5.0248, 25.73) ccw
  line L3349 (11.4808, 27.48) -> (11.9888, 27.48)
  arc A2183 (11.7348, 27.2768) -> (11.7348, 27.6832) centre (11.7348, 27.48) ccw
  line L3350 (4.7708, 25.73) -> (5.2788, 25.73)
  arc A2184 (12.0523, 27.48) -> (11.4173, 27.48) centre (11.7348, 27.48) ccw
  arc A2185 (11.7348, 27.6832) -> (11.7348, 27.2768) centre (11.7348, 27.48) ccw
  arc A2186 (5.0248, 25.1395) -> (5.0248, 26.3206) centre (5.0248, 25.73) ccw
  line L3351 (4.7708, 37.77) -> (5.2788, 37.77)
  arc A2187 (11.4173, 27.48) -> (12.0523, 27.48) centre (11.7348, 27.48) ccw
  line L3352 (4.7708, 37.77) -> (5.2788, 37.77)
  line L3353 (11.7348, 27.734) -> (11.7348, 27.226)
  arc A2188 (12.0523, 27.48) -> (11.4173, 27.48) centre (11.7348, 27.48) ccw
  arc A2189 (5.0248, 26.3206) -> (5.0248, 25.1395) centre (5.0248, 25.73) ccw
  arc A2190 (5.0248, 37.1794) -> (5.0248, 38.3605) centre (5.0248, 37.77) ccw
  arc A2191 (4.1358, 25.73) -> (5.9138, 25.73) centre (5.0248, 25.73) ccw
  line L3354 (5.0248, 38.024) -> (5.0248, 37.516)
  arc A2192 (5.0248, 37.1794) -> (5.0248, 38.3605) centre (5.0248, 37.77) ccw
  line L3355 (4.7708, 37.77) -> (5.2788, 37.77)
  line L3356 (5.0248, 38.024) -> (5.0248, 37.516)
  line L3357 (5.0248, 25.984) -> (5.0248, 25.476)
  arc A2193 (4.1358, 25.73) -> (5.9138, 25.73) centre (5.0248, 25.73) ccw
  arc A2194 (4.1358, 25.73) -> (5.9138, 25.73) centre (5.0248, 25.73) ccw
  line L3358 (4.7708, 37.77) -> (5.2788, 37.77)
  arc A2195 (5.0248, 37.1794) -> (5.0248, 38.3605) centre (5.0248, 37.77) ccw
  line L3359 (70.597, 47.309) -> (70.597, 47.989)
  line L3360 (15.81, 31.46) -> (14.81, 31.46)
  line L3361 (70.247, 47.649) -> (72.247, 47.649)
  line L3362 (70.597, 47.309) -> (70.597, 47.989)
  line L3363 (72.247, 50.649) -> (70.247, 50.649)
  arc A2196 (5.9138, 37.77) -> (4.1358, 37.77) centre (5.0248, 37.77) ccw
  arc A2197 (5.0248, 37.1794) -> (5.0248, 38.3605) centre (5.0248, 37.77) ccw
  line L3364 (4.7708, 37.77) -> (5.2788, 37.77)
  line L3365 (14.535, 30.66) -> (15.21, 30.66)
  arc A2198 (14.1876, 31.5856) -> (14.5876, 31.5856) centre (14.3876, 31.5856) ccw
  line L3366 (14.81, 28.86) -> (15.81, 28.86)
  line L3367 (71.247, 47.309) -> (71.247, 47.989)
  line L3368 (15.41, 29.66) -> (16.085, 29.66)
  line L3369 (71.897, 47.309) -> (71.897, 47.989)
  line L3370 (71.897, 47.309) -> (71.897, 47.989)
  line L3371 (5.0248, 38.024) -> (5.0248, 37.516)
  arc A2199 (5.9138, 37.77) -> (4.1358, 37.77) centre (5.0248, 37.77) ccw
  arc A2200 (4.1358, 37.77) -> (5.9138, 37.77) centre (5.0248, 37.77) ccw
  arc A2201 (4.1358, 37.77) -> (5.9138, 37.77) centre (5.0248, 37.77) ccw
  line L3372 (14.535, 30.66) -> (15.21, 30.66)
  arc A2202 (5.9138, 37.77) -> (4.1358, 37.77) centre (5.0248, 37.77) ccw
  line L3373 (5.0248, 38.024) -> (5.0248, 37.516)
  line L3374 (14.535, 31.16) -> (15.21, 31.16)
  line L3375 (14.535, 29.66) -> (15.21, 29.66)
  line L3376 (15.41, 29.16) -> (16.085, 29.16)
  arc A2203 (14.5876, 31.5856) -> (14.1876, 31.5856) centre (14.3876, 31.5856) ccw
  line L3377 (14.535, 29.16) -> (15.21, 29.16)
  line L3378 (71.897, 50.309) -> (71.897, 50.989)
  arc A2204 (4.1358, 37.77) -> (5.9138, 37.77) centre (5.0248, 37.77) ccw
  line L3379 (15.41, 31.16) -> (16.085, 31.16)
  line L3380 (71.897, 47.309) -> (71.897, 47.989)
  line L3381 (5.0248, 38.024) -> (5.0248, 37.516)
  line L3382 (71.247, 47.309) -> (71.247, 47.989)
  line L3383 (15.41, 29.66) -> (16.085, 29.66)
  line L3384 (14.535, 30.16) -> (15.21, 30.16)
  line L3385 (15.41, 31.16) -> (16.085, 31.16)
  line L3386 (70.247, 50.649) -> (70.247, 47.649)
  line L3387 (70.597, 47.309) -> (70.597, 47.989)
  arc A2205 (70.2222, 47.2028) -> (70.2222, 46.8028) centre (70.2222, 47.0028) ccw
  arc A2206 (5.0248, 37.1794) -> (5.0248, 38.3605) centre (5.0248, 37.77) ccw
  line L3388 (5.0248, 38.024) -> (5.0248, 37.516)
  arc A2207 (5.0248, 38.3605) -> (5.0248, 37.1794) centre (5.0248, 37.77) ccw
  arc A2208 (4.1358, 37.77) -> (5.9138, 37.77) centre (5.0248, 37.77) ccw
  line L3389 (5.0248, 38.024) -> (5.0248, 37.516)
  line L3390 (14.535, 29.66) -> (15.21, 29.66)
  line L3391 (14.535, 30.16) -> (15.21, 30.16)
  arc A2209 (5.0248, 37.1794) -> (5.0248, 38.3605) centre (5.0248, 37.77) ccw
  line L3392 (14.535, 29.66) -> (15.21, 29.66)
  arc A2210 (5.9138, 37.77) -> (4.1358, 37.77) centre (5.0248, 37.77) ccw
  line L3393 (15.81, 28.86) -> (15.81, 31.46)
  line L3394 (14.535, 31.16) -> (15.21, 31.16)
  line L3395 (4.7708, 37.77) -> (5.2788, 37.77)
  arc A2211 (4.1358, 37.77) -> (5.9138, 37.77) centre (5.0248, 37.77) ccw
  arc A2212 (5.9138, 37.77) -> (4.1358, 37.77) centre (5.0248, 37.77) ccw
  line L3396 (14.81, 31.46) -> (14.81, 28.86)
  line L3397 (14.535, 30.66) -> (15.21, 30.66)
  line L3398 (14.535, 29.16) -> (15.21, 29.16)
  line L3399 (15.41, 29.16) -> (16.085, 29.16)
  line L3400 (14.535, 31.16) -> (15.21, 31.16)
  line L3401 (14.535, 30.16) -> (15.21, 30.16)
  line L3402 (14.535, 29.16) -> (15.21, 29.16)
  line L3403 (4.7708, 37.77) -> (5.2788, 37.77)
  line L3404 (15.41, 29.16) -> (16.085, 29.16)
  line L3405 (72.247, 47.649) -> (72.247, 50.649)
  line L3406 (70.597, 50.309) -> (70.597, 50.989)
  line L3407 (77.967, 58.539) -> (77.117, 58.539)
  arc A2213 (74.549, 57.023) -> (74.549, 56.515) centre (74.549, 56.769) ccw
  line L3408 (77.842, 57.1015) -> (77.242, 57.1015)
  line L3409 (76.2545, 55.889) -> (76.2545, 56.489)
  line L3410 (15.41, 30.16) -> (16.085, 30.16)
  arc A2214 (77.242, 57.6015) -> (77.242, 57.4765) centre (77.242, 57.539) ccw
  line L3411 (76.1295, 56.489) -> (76.1295, 55.889)
  arc A2215 (76.7545, 56.489) -> (76.6295, 56.489) centre (76.692, 56.489) ccw
  arc A2216 (76.1295, 55.889) -> (76.2545, 55.889) centre (76.192, 55.889) ccw
  arc A2217 (77.842, 56.9765) -> (77.842, 57.1015) centre (77.842, 57.039) ccw
  arc A2218 (73.914, 55.499) -> (73.914, 54.991) centre (73.914, 55.245) ccw
  arc A2219 (74.549, 56.515) -> (74.549, 57.023) centre (74.549, 56.769) ccw
  line L3412 (74.7545, 55.889) -> (74.7545, 56.489)
  line L3413 (15.41, 31.16) -> (16.085, 31.16)
  arc A2220 (75.6295, 55.889) -> (75.7545, 55.889) centre (75.692, 55.889) ccw
  line L3414 (15.41, 30.16) -> (16.085, 30.16)
  arc A2221 (76.2545, 56.489) -> (76.1295, 56.489) centre (76.192, 56.489) ccw
  line L3415 (15.41, 30.66) -> (16.085, 30.66)
  line L3416 (76.6295, 56.489) -> (76.6295, 55.889)
  line L3417 (75.192, 55.764) -> (75.192, 56.614)
  line L3418 (77.692, 56.039) -> (77.692, 60.039)
  line L3419 (15.41, 30.66) -> (16.085, 30.66)
  arc A2222 (77.242, 58.1015) -> (77.242, 57.9765) centre (77.242, 58.039) ccw
  line L3420 (77.967, 57.539) -> (77.117, 57.539)
  line L3421 (15.41, 30.66) -> (16.085, 30.66)
  line L3422 (71.247, 48.299) -> (71.247, 49.999)
  arc A2223 (77.842, 57.9765) -> (77.842, 58.1015) centre (77.842, 58.039) ccw
  line L3423 (77.967, 57.039) -> (77.117, 57.039)
  line L3424 (71.247, 50.309) -> (71.247, 50.989)
  arc A2224 (75.2545, 56.489) -> (75.1295, 56.489) centre (75.192, 56.489) ccw
  line L3425 (75.692, 55.764) -> (75.692, 56.614)
  line L3426 (71.247, 48.299) -> (71.247, 49.999)
  line L3427 (73.692, 60.039) -> (73.692, 56.039)
  line L3428 (15.41, 29.66) -> (16.085, 29.66)
  line L3429 (71.247, 50.309) -> (71.247, 50.989)
  arc A2225 (74.6295, 55.889) -> (74.7545, 55.889) centre (74.692, 55.889) ccw
  line L3430 (15.41, 30.16) -> (16.085, 30.16)
  line L3431 (75.1295, 56.489) -> (75.1295, 55.889)
  line L3432 (75.192, 55.764) -> (75.192, 56.614)
  arc A2226 (75.1295, 55.889) -> (75.2545, 55.889) centre (75.192, 55.889) ccw
  line L3433 (70.597, 50.309) -> (70.597, 50.989)
  line L3434 (75.692, 55.764) -> (75.692, 56.614)
  line L3435 (77.692, 60.039) -> (73.692, 60.039)
  line L3436 (74.6295, 56.489) -> (74.6295, 55.889)
  arc A2227 (74.7545, 56.489) -> (74.6295, 56.489) centre (74.692, 56.489) ccw
  line L3437 (71.897, 50.309) -> (71.897, 50.989)
  line L3438 (75.2545, 55.889) -> (75.2545, 56.489)
  line L3439 (77.967, 57.539) -> (77.117, 57.539)
  line L3440 (74.692, 55.764) -> (74.692, 56.614)
  line L3441 (76.192, 55.764) -> (76.192, 56.614)
  arc A2228 (70.2222, 46.8028) -> (70.2222, 47.2028) centre (70.2222, 47.0028) ccw
  line L3442 (71.897, 50.309) -> (71.897, 50.989)
  line L3443 (73.692, 56.039) -> (77.692, 56.039)
  arc A2229 (75.7545, 56.489) -> (75.6295, 56.489) centre (75.692, 56.489) ccw
  line L3444 (75.6295, 56.489) -> (75.6295, 55.889)
  line L3445 (77.242, 56.9765) -> (77.842, 56.9765)
  line L3446 (71.247, 47.309) -> (71.247, 47.989)
  line L3447 (70.597, 50.309) -> (70.597, 50.989)
  line L3448 (75.7545, 55.889) -> (75.7545, 56.489)
  arc A2230 (73.914, 54.991) -> (73.914, 55.499) centre (73.914, 55.245) ccw
  line L3449 (71.247, 48.299) -> (71.247, 49.999)
  line L3450 (74.692, 55.764) -> (74.692, 56.614)
  line L3451 (71.247, 50.309) -> (71.247, 50.989)
  arc A2231 (75.2545, 60.189) -> (75.1295, 60.189) centre (75.192, 60.189) ccw
  arc A2232 (77.242, 57.1015) -> (77.242, 56.9765) centre (77.242, 57.039) ccw
  arc A2233 (75.6295, 59.589) -> (75.7545, 59.589) centre (75.692, 59.589) ccw
  arc A2234 (76.7545, 60.189) -> (76.6295, 60.189) centre (76.692, 60.189) ccw
  arc A2235 (74.7545, 60.189) -> (74.6295, 60.189) centre (74.692, 60.189) ccw
  line L3452 (77.242, 57.4765) -> (77.842, 57.4765)
  line L3453 (75.2545, 59.589) -> (75.2545, 60.189)
  line L3454 (74.142, 58.6015) -> (73.542, 58.6015)
  line L3455 (74.267, 58.539) -> (73.417, 58.539)
  line L3456 (76.692, 59.464) -> (76.692, 60.314)
  line L3457 (76.7545, 55.889) -> (76.7545, 56.489)
  line L3458 (77.242, 57.9765) -> (77.842, 57.9765)
  line L3459 (77.842, 59.1015) -> (77.242, 59.1015)
  arc A2236 (73.542, 59.1015) -> (73.542, 58.9765) centre (73.542, 59.039) ccw
  line L3460 (74.267, 59.039) -> (73.417, 59.039)
  line L3461 (77.967, 58.039) -> (77.117, 58.039)
  line L3462 (74.267, 59.039) -> (73.417, 59.039)
  line L3463 (75.192, 59.464) -> (75.192, 60.314)
  line L3464 (75.192, 59.464) -> (75.192, 60.314)
  line L3465 (74.692, 59.464) -> (74.692, 60.314)
  line L3466 (75.1295, 60.189) -> (75.1295, 59.589)
  arc A2237 (76.1295, 59.589) -> (76.2545, 59.589) centre (76.192, 59.589) ccw
  arc A2238 (77.842, 57.4765) -> (77.842, 57.6015) centre (77.842, 57.539) ccw
  line L3467 (75.692, 59.464) -> (75.692, 60.314)
  arc A2239 (76.6295, 59.589) -> (76.7545, 59.589) centre (76.692, 59.589) ccw
  arc A2240 (74.142, 58.9765) -> (74.142, 59.1015) centre (74.142, 59.039) ccw
  line L3468 (77.967, 57.039) -> (77.117, 57.039)
  arc A2241 (76.2545, 60.189) -> (76.1295, 60.189) centre (76.192, 60.189) ccw
  arc A2242 (77.242, 59.1015) -> (77.242, 58.9765) centre (77.242, 59.039) ccw
  line L3469 (75.692, 59.464) -> (75.692, 60.314)
  arc A2243 (74.6295, 59.589) -> (74.7545, 59.589) centre (74.692, 59.589) ccw
  line L3470 (77.842, 58.6015) -> (77.242, 58.6015)
  arc A2244 (77.842, 58.4765) -> (77.842, 58.6015) centre (77.842, 58.539) ccw
  line L3471 (76.7545, 59.589) -> (76.7545, 60.189)
  line L3472 (80.785, 49.954) -> (80.785, 50.904)
  line L3473 (76.1295, 60.189) -> (76.1295, 59.589)
  line L3474 (74.7545, 59.589) -> (74.7545, 60.189)
  line L3475 (76.192, 59.464) -> (76.192, 60.314)
  arc A2245 (77.242, 58.6015) -> (77.242, 58.4765) centre (77.242, 58.539) ccw
  line L3476 (77.967, 59.039) -> (77.117, 59.039)
  line L3477 (73.542, 58.9765) -> (74.142, 58.9765)
  line L3478 (77.967, 59.039) -> (77.117, 59.039)
  arc A2246 (77.842, 58.9765) -> (77.842, 59.1015) centre (77.842, 59.039) ccw
  line L3479 (77.842, 57.6015) -> (77.242, 57.6015)
  line L3480 (77.967, 58.539) -> (77.117, 58.539)
  line L3481 (77.842, 58.1015) -> (77.242, 58.1015)
  line L3482 (77.242, 58.4765) -> (77.842, 58.4765)
  line L3483 (75.6295, 60.189) -> (75.6295, 59.589)